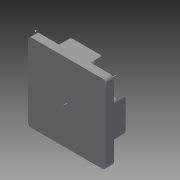
# Autodesk Inventor part: endcap_2020_new
Saved by Autodesk Inventor 2015 (Build 190159000, 159)
## iProperties
Created: 2015-09-19
Part Number: endcap_2020_new
Material: Generic
Document SubType Name: Modeling
Designer: Erwin
Density: 1 g/cm^3
Appearance: Default
Author: Erwin
Autodesk Inventor part; units mm, degrees
ref_plane "YZ Plane" through (0, 0, 0) normal (1, 0, 0) x (0, 1, 0)
ref_plane "XZ Plane" through (0, 0, 0) normal (0, 1, 0) x (-1, 0, 0)
ref_plane "XY Plane" through (0, 0, 0) normal (0, 0, 1) x (1, 0, 0)
sketch "Sketch1" plane through (0, 0, 0) normal (0, 1, 0) x (-1, 0, 0)
  line L0 (0, 0) -> (-20, 0)
  line L1 (-20, 0) -> (-20, -20)
  line L2 (-20, -20) -> (0, -20)
  line L3 (0, -20) -> (0, 0)
  dimension "d0" = 20
  dimension "d1" = 20
  constraints: 8 end point, 2 parallel, 1 horizontal, 1 perpendicular
  measures "d0" distance of L2.end L1.end
  measures "d1" distance of L1.end L0.end
extrude "Extrusion1" add sketch "Sketch1" along normal blind 2
sketch "Sketch2" plane through (0, 2, 0) normal (0, 1, 0) x (1, 0, 0)
  line L0 (0, 20) -> (0, 0) construction
  line L1 (20, 0) -> (20, 20) construction
  line L2 (0, 10) -> (0, 14)
  line L3 (0, 10) -> (5.5, 10) construction
  line L4 (0, 10) -> (1.8, 10) construction
  line L5 (1.8, 10) -> (1.8, 19.4431) construction
  line L6 (0, 14) -> (1.8, 12.2)
  line L7 (0, 14) -> (2.5456, 14) construction
  line L8 (1.8, 12.2) -> (1.8, 14)
  line L9 (1.8, 14) -> (5.5, 10)
  line L10 (0, 0) -> (0, 20) construction
  line L11 (0, 10) -> (0, 6)
  line L12 (1.8, 10) -> (1.8, 0.5569) construction
  line L13 (0, 6) -> (1.8, 7.8)
  line L14 (1.8, 7.8) -> (1.8, 6)
  line L15 (1.8, 6) -> (5.5, 10)
  dimension "d4" = 4
  dimension "d5" = 5.5
  dimension "d6" = 1.8
  dimension "d7" = 45
  constraints: 28 end point, 8 point on line, 6 symmetric about line, 2 horizontal, 1 equal length, 1 midpoint, 1 perpendicular
  measures "d4" distance of L2.start L2.end
  measures "d5" distance of L2.start L3.end
  measures "d6" distance of L2.start L4.end
  measures "d7" angle of L6 L7
extrude "Extrusion2" add sketch "Sketch2" along normal blind 3
fillet "Fillet1" radius 1 3 edges at (5.5, 3.5, -10) (1.8, 3.5, -6) (1.8, 3.5, -14)
fillet "Fillet2" radius 1 4 edges at (0, 1, 0) (20, 1, 0) (20, 1, -20) (0, 1, -20)
fillet "Fillet3" radius 0.4 7 edges at (2.5522, 5, -12.6325) (5.1378, 5, -10) (4.1156, 5, -8.5034) (2.5522, 5, -7.3675) (4.1156, 5, -11.4966) (0.9, 5, -13.1) (0.9, 5, -6.9)
sketch "Sketch3" plane through (0, 2, 0) normal (0, 1, 0) x (1, 0, 0)
  point P0 (0, 0)
  point P1 (10, 10)
pattern_circular "Circular Pattern1" count 4 over 360 about axis through (10, 2, -10) along (0, 1, 0) of "Fillet1", "Extrusion2", "Fillet3"
body "Solid1"
